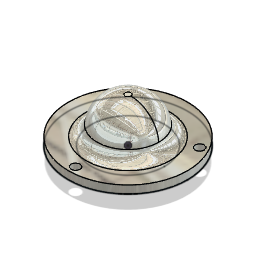
RollerBack_New (Autodesk Fusion 360 archive; units mm, degrees)
design "RollerBacl"
Autodesk Fusion 360 part; units mm, degrees
sketch "Sketch1" plane through (0, 0, 0) normal (0, 1, 0) x (1, 0, 0)
  circle A0 centre (0, 0) radius 13
  circle A1 centre (0, 0) radius 21.25
  dimension "d1" = 26
  dimension "d2" = 42.5
  constraint coincident A0.centre A1.centre
  measures "d1" diameter of A0
  measures "d2" diameter of A1
extrude "Extrude1" add sketch "Sketch1" against normal blind 5 contours A0
extrude "Extrude2" add sketch "Sketch1" along normal blind 2.8 contours A0 | A1
sketch "Sketch2" plane through (0, 2.8, 0) normal (0, 1, 0) x (-1, 0, 0)
  circle A0 centre (0, 0) radius 21.25
  circle A1 centre (0, 0) radius 11
  dimension "d7" = 22
  constraint coincident A0.centre A1.centre
  measures "d7" diameter of A1
extrude "Extrude3" add sketch "Sketch2" along normal blind 13 contours A1
fillet "Fillet1" radius 4 1 edges at (10.2556, 2.8, 3.9778)
fillet "Fillet2" radius 10 1 edges at (10.2556, 15.8, -3.9778)
fillet "Fillet3" radius 2 1 edges at (-12.1203, 0, 4.701)
fillet "Fillet4" radius 2 1 edges at (-12.1203, -5, -4.701)
sketch "Sketch3" plane through (0, 2.8, 0) normal (0, 1, 0) x (-1, 0, 0)
  circle A0 centre (0, 0) radius 21.25
  circle A1 centre (0, 0) radius 15
  circle A2 centre (0, 0) radius 18.75
  circle A3 centre (0, 18.75) radius 1.6
  circle A4 centre (-16.238, -9.375) radius 1.6
  circle A5 centre (16.238, -9.375) radius 1.6
  dimension "d18" = 37.5
  dimension "d19" = 3.2
  dimension "d21" = 360
  constraint coincident A0.centre A1.centre
  constraint coincident A2 A3.centre
  measures "d18" diameter of A2
  measures "d19" diameter of A3
extrude "Extrude4" cut sketch "Sketch3" against normal blind 5 contours A2 A3 | A2 A3 | A2 A5 | A2 A5 | A2 A4 | A2 A4
equation "d18 = 42.500 mm - 5 mm"
